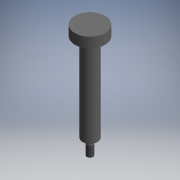
# Autodesk Inventor part: ESBF-BS-100-100-20P---(KS_0)
Saved by Autodesk Inventor 2017.3 (Build 213256000, 256)
## iProperties
Part Number: ESBF-BS-100-100-20P---(KS_0)
Material: Generic
Catalog Web Link: www.cadenas.de
Description: ESBF-(KS)-Electro-cylinder
Vendor: FESTO
Document SubType Name: Modeling
Designer: partserver
Manufacturer: FESTO
Mass: 851.947 g
Surface Area: 752.864 cm^2
Volume: 851.947 cm^3
Density: 1 g/cm^3
Appearance: PSOLRGB-128-128-128
Category: PARTsolutions
Company: FESTO
Title: ESBF-BS-100-100-20P---(KS_0)
Author: Cadenas PARTsolutions
Comments: Electro-cylinder
PSOL_IDENT_0: {$CADENAS_DATA\23d-libs\festo\parts\e\esbf\parts\esbf_ks.prj},235 {VTYP=3D},{NB=ESBF-BS-100-100-20P-
PSOL_IDENT_1: --(KS_0)},{LINA=ESBF-BS-100-100-20P---(KS_0)},{NN=ESBF-(KS)},{DATE=13.05.2020 13:32:49},{GEOMDATE=17
PSOL_IDENT_2: .03.2017 10:52:53},{VERSION=},{LINEID=30},{WBVAR=HUB,SPI,KOL,KOLE,HUBST},{WBNUMERIC=HUB,KOLE,HUBST}
PSOL_IDENT_3: {NB=ESBF-BS-100-100-20P---(KS_0)},{LINA=ESBF-BS-100-100-20P---(KS_0)},{KT=DUMMY},{TNR=574092},{TYP=
PSOL_IDENT_4: ESBF-BS-100},{KDM=100},{HUB=100},{HUBMAX=1500},{SPI=20P},{KOL=-},{KOLT=},{KOLE=0},{KOLET=},{HUBST=0}
PSOL_IDENT_5: ,{A2=0},{AM=40.000},{WH=51.000},{L1=34.000},{L2=224.000},{L3=39.500},{L4=30.000},{L5=6.100},{L7=11.0
PSOL_IDENT_6: 00},{G=39.000},{G1=39.000},{VA=12.000},{ZJ=275.000},{KK=20.000},{KKP=1.500},{MM=25.000},{D1=50.000},
PSOL_IDENT_7: {D2=24.000},{D4=13.000},{SW1=22.000},{K1=12.000},{K1T=20.000},{X=10.000}
NB: ESBF-BS-100-100-20P---(KS_0)
NN: ESBF-(KS)
NT: Electro-cylinder
NBSYN: $TYP.-$HUB.-$SPI.$KOLT.$KOLET.---(KS_$HUBST.)
LINA: ESBF-BS-100-100-20P---(KS_0)
CATALOG: Festo
TNR: 574092
TYP: ESBF-BS-100
KDM: 100
HUB: 100
HUBMAX: 1500
SPI: 20P
KOL: -
KOLE: 0
HUBST: 0
AM: 40
WH: 51
L1: 34
L2: 224
L3: 39.5
L4: 30
L5: 6.1
L7: 11
G: 39
G1: 39
VA: 12
ZJ: 275
KK: 20
KKP: 1.5
MM: 25
D1: 50
D2: 24
D4: 13
SW1: 22
K1: 12
K1T: 20
X: 10
SUPPLIER: FESTO
ARTICLENO: ESBF-BS-100-100-20P---(KS_0)
BOMINFO: ESBF-BS-100-100-20P---(KS_0)
CREATOR: CADENAS GmbH
Autodesk Inventor part; units mm, degrees
sketch "Sketch_1" plane through (0, 0, 0) normal (1, 0, 0) x (0, 1, 0)
  line L0 (0, -285) -> (0, 51)
  line L1 (0, 51) -> (12, 51)
  line L2 (12, 51) -> (12.5, 50.5)
  line L3 (12.5, 50.5) -> (12.5, 40)
  line L4 (12.5, 40) -> (24.4226, 40)
  line L5 (24.4226, 40) -> (25, 39)
  line L6 (25, 39) -> (25, -251.6667)
  line L7 (25, -251.6667) -> (50, -251.6667)
  line L8 (50, -251.6667) -> (50, -285)
  line L9 (50, -285) -> (0, -285)
  line L10 (0, -285) -> (0, 51)
  constraints: 22 end point
revolve "Revolution1" add sketch "Sketch_1" angle 360 about axis through (0, 0, -285) along (0, 0, -1)
sketch "Sketch_3" plane through (0, 0, 0) normal (0, 1, 0) x (-1, 0, 0)
  line L0 (14, 41) -> (14, 54)
  line L1 (14, 54) -> (-14, 54)
  line L2 (-14, 54) -> (-14, 41)
  line L3 (-14, 41) -> (-11, 41)
  line L4 (-11, 41) -> (-11, 51)
  line L5 (-11, 51) -> (11, 51)
  line L6 (11, 51) -> (11, 41)
  line L7 (11, 41) -> (14, 41)
  constraints: 16 end point
extrude "Extrusion1" cut sketch "Sketch_3" along normal mid plane 50
sketch "Sketch_2" plane through (0, 0, 0) normal (1, 0, 0) x (0, 1, 0)
  line L0 (0, 51) -> (0, 91)
  line L1 (0, 91) -> (9.08, 91)
  line L2 (9.08, 91) -> (10, 90.08)
  line L3 (10, 90.08) -> (10, 54.92)
  line L4 (10, 54.92) -> (9.08, 54)
  line L5 (9.08, 54) -> (9.08, 51.6)
  arc A0 (9.08, 51.6) -> (9.68, 51) centre (9.68, 51.6) ccw
  line L6 (9.68, 51) -> (0, 51)
  line L7 (0, 51) -> (0, 91)
  constraints: 16 end point, 2 point on circle, 1 centre point
revolve "Revolution2" add sketch "Sketch_2" angle 360 about axis through (0, 0, 51) along (0, 0, -1)
thread "Thread1" size "M20x1.5" class "6g" standard "ISO Metric profile" full length
ref_plane "ANBAU_XY" through (0, 0, -285) normal (0, 0, -1) x (1, 0, 0)
ref_plane "ANBAU_YZ" through (0, 0, -285) normal (1, 0, 0) x (0, -1, 0)
ref_plane "ANBAU_ZX" through (0, 0, -285) normal (0, -1, 0) x (0, 0, -1)
ref_plane "NUT_XY" through (0, 0, 61) normal (0, 0, -1) x (1, 0, 0)
ref_plane "NUT_YZ" through (0, 0, 61) normal (1, 0, 0) x (0, -1, 0)
ref_plane "NUT_ZX" through (0, 0, 61) normal (0, -1, 0) x (0, 0, -1)
body "Solid1"
